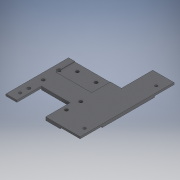
# Autodesk Inventor part: SUPPORT MAIN FRAME MOTOR-BALL SCREW-REV-B
Saved by Autodesk Inventor 2018 (Build 220112000, 112)
## iProperties
Created: 2018-03-20
Part Number: SUPPORT MAIN FRAME MOTOR-BALL SCREW-REV-B
Material: Steel
Document SubType Name: Modeling
Designer: M224826
Density: 7.85 g/cm^3
Appearance: Iron - Cast
Author: M224826
Autodesk Inventor part; units mm, degrees
ref_plane "YZ Plane" through (0, 0, 0) normal (1, 0, 0) x (0, 1, 0)
ref_plane "XZ Plane" through (0, 0, 0) normal (0, 1, 0) x (-1, 0, 0)
ref_plane "XY Plane" through (0, 0, 0) normal (0, 0, 1) x (1, 0, 0)
sketch "Sketch1" plane through (0, 0, 0) normal (0, 0, 1) x (1, 0, 0)
  circle A0 centre (60, -12) radius 5
  line L0 (0, 0) -> (0, 90) construction
  circle A1 centre (-60, -12) radius 5
  line L1 (46, -32) -> (-46, -32)
  line L2 (-46, -32) -> (-46, -110)
  line L3 (-46, -110) -> (-81, -110)
  line L4 (-81, 90) -> (88, 90)
  line L5 (88, 90) -> (88, 190)
  line L6 (88, 190) -> (156, 190)
  line L7 (156, 190) -> (156, -110)
  line L8 (156, -110) -> (46, -110)
  line L9 (46, -110) -> (46, -32)
  line L10 (-81, -110) -> (-81, 90)
  circle A2 centre (30, 67) radius 5
  circle A3 centre (-30, 67) radius 5
  circle A4 centre (60, -58) radius 5
  circle A5 centre (-60, -58) radius 5
  circle A6 centre (-61, -85) radius 4.25
  circle A7 centre (140, -80) radius 4.25
  circle A8 centre (137, 152) radius 4.25
  circle A9 centre (-61, 40) radius 4.25
  point P0 (0, -32)
  dimension "d82" = 10
  dimension "d83" = 60
  dimension "d86" = 32
  dimension "d87" = 90
  dimension "d88" = 92
  dimension "d90" = 300
  dimension "d91" = 200
  dimension "d92" = 35
  dimension "d93" = 68
  dimension "d94" = 100
  dimension "d95" = 237
  dimension "d96" = 79
  dimension "d98" = 60
  dimension "d100" = 46
  dimension "d101" = 8.5
  dimension "d102" = 140
  dimension "d103" = 80
  dimension "d104" = 3
  dimension "d105" = 152
  dimension "d106" = 61
  dimension "d107" = 85
  dimension "d108" = 40
  dimension "d136" = 12
  constraints: 22 end point, 10 centre point, 6 equal radius, 6 perpendicular, 4 vertical alignment, 3 point on line, 1 horizontal, 1 horizontal alignment, 1 midpoint, 1 symmetric about line, 1 vertical, 2 other
  measures "d82" diameter of A0
  measures "d83" horizontal distance of A0.centre L0.start
  measures "d86" distance from line of L1 L0.start
  measures "d87" distance from line of L0.start L4
  measures "d88" distance of L1.start L1.end
  measures "d90" distance of L6.end L7.end
  measures "d91" distance of L3.end L4.start
  measures "d92" distance of L2.end L3.end
  measures "d93" distance of L5.end L6.end
  measures "d94" distance of L4.end L5.end
  measures "d95" distance between parallel lines of L7 L10
  measures "d96" vertical distance of A2.centre A0.centre
  measures "d98" distance of A2.centre A3.centre
  measures "d100" distance of A5.centre A1.centre
  measures "d101" diameter of A7
  measures "d102" horizontal distance of A7.centre L0.start
  measures "d103" vertical distance of L0.start A7.centre
  measures "d104" horizontal distance of A8.centre A7.centre
  measures "d105" vertical distance of A8.centre L0.start
  measures "d106" horizontal distance of A6.centre L0.start
  measures "d107" vertical distance of A6.centre L0.start
  measures "d108" vertical distance of A9.centre L0.start
  measures "d136" vertical distance of A0.centre L0.start
extrude "Extrusion1" add sketch "Sketch1" along normal blind 10
sketch "Sketch2" plane through (0, 0, 10) normal (0, 0, 1) x (1, 0, 0)
  line L0 (-81, 90) -> (88, 90) projected
  line L1 (-61, 90) -> (53, 90)
  line L2 (53, 90) -> (53, 30)
  line L3 (53, 30) -> (-61, 30)
  line L4 (-61, 30) -> (-61, 90)
  line L5 (-81, 90) -> (-81, -110) projected
  point P0 (0, 0)
  dimension "d111" = 114
  dimension "d112" = 60
  dimension "d113" = 20
  constraints: 8 end point, 2 parallel, 1 horizontal, 1 perpendicular, 1 point on line
  measures "d111" distance of L2.end L3.end
  measures "d112" distance of L1.end L2.end
  measures "d113" distance between parallel lines of L4 L5
extrude "Extrusion2" cut sketch "Sketch2" against normal blind 1.5
sketch "Sketch3" plane through (0, 0, 8.5) normal (0, 0, 1) x (1, 0, 0)
  circle A0 centre (-61, 40) radius 4.25 projected
  circle A1 centre (-61, 40) radius 7
  point P0 (0, 0)
  dimension "d116" = 14
  constraints: 1 centre point, 1 coincident
  measures "d116" diameter of A1
extrude "Extrusion3" cut sketch "Sketch3" along normal up to surface (1.5 mm away)
thread "Thread1" size "M10x1.5" class "6H" standard "ISO Metric profile" full length
thread "Thread2" size "M10x1.5" class "6H" standard "ANSI Metric M Profile" full length
thread "Thread3" size "M10x1.5" class "6H" standard "ANSI Metric M Profile" full length
thread "Thread4" size "M10x1.5" class "6H" standard "ANSI Metric M Profile" full length
sketch "Sketch4" plane through (0, 0, 0) normal (0, 0, -1) x (-1, 0, 0)
  line L0 (-156, 190) -> (-156, -110) projected
  line L1 (-156, 190) -> (-90, 190)
  line L2 (-88, 190) -> (-156, 190) projected
  line L3 (-90, 190) -> (-90, 128)
  line L4 (-88, 90) -> (-88, 190) projected
  line L5 (-90, 190) -> (-28, 190) construction
  line L6 (-90, 128) -> (-156, 128)
  line L7 (-156, 128) -> (-156, 190)
  line L8 (-156, -110) -> (-46, -110) projected
  line L9 (-156, -110) -> (-92, -110)
  line L10 (-92, -110) -> (-92, -39.5)
  line L11 (-92, -39.5) -> (-156, -39.5)
  line L12 (81, -110) -> (81, 90) projected
  line L13 (46, -32) -> (46, -110) projected
  line L14 (81, -110) -> (46, -110)
  line L15 (46, -110) -> (46, 90)
  line L16 (81, 90) -> (-88, 90) projected
  point P0 (0, 0)
  dimension "d127" = 66
  dimension "d128" = 62
  dimension "d129" = 90
  dimension "d130" = 66
  dimension "d131" = 90
  dimension "d134" = 64
  dimension "d135" = 70.5
  constraints: 20 end point, 5 perpendicular, 4 point on line, 2 horizontal, 1 parallel
  measures "d127" distance of L0.start L1.end
  measures "d128" distance of L1.end L3.end
  measures "d129" angle of L3 L5
  measures "d130" distance of L3.end L6.end
  measures "d131" angle of L3 L6
  measures "d134" distance of L0.end L9.end
  measures "d135" distance of L9.end L10.end
extrude "Extrusion4" cut sketch "Sketch4" against normal blind 4
body "Solid1"
